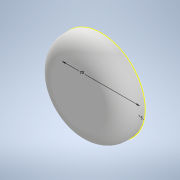
# Autodesk Inventor part: Top_and_Bottom
Saved by Autodesk Inventor 2020.2 (Build 242310000, 310)
## iProperties
Created: 2020-03-04
Part Number: Top_and_Bottom
Material: Generic
Document SubType Name: Modeling
Designer: linus
Density: 1 g/cm^3
Appearance: Default
Author: linus
Autodesk Inventor part; units mm, degrees
ref_plane "YZ Plane" through (0, 0, 0) normal (1, 0, 0) x (0, 1, 0)
ref_plane "XZ Plane" through (0, 0, 0) normal (0, 1, 0) x (-1, 0, 0)
ref_plane "XY Plane" through (0, 0, 0) normal (0, 0, 1) x (1, 0, 0)
sketch "Sketch1" plane through (0, 0, 0) normal (0, 1, 0) x (-1, 0, 0)
  line L0 (0, 0) -> (-40, 0)
  line L1 (-40, 0) -> (-40, 20)
  line L2 (-40, 20) -> (0, 20)
  line L3 (0, 20) -> (0, 0)
  dimension "d0" = 40
  dimension "d1" = 20
  constraints: 8 end point, 2 parallel, 1 horizontal, 1 perpendicular
  measures "d0" distance of L1.end L2.end
  measures "d1" distance of L0.end L1.end
revolve "Revolution1" add sketch "Sketch1" angle 360 about axis through (40, 0, 0) along (0, 0, 1)
fillet "Fillet1" radius 15 1 edges at (80, 0, 20)
sketch "Sketch2" plane through (40, 0, 0) normal (0, 0, -1) x (-1, 0, 0)
  circle A0 centre (0, 0) radius 35
  circle A1 centre (0, 0) radius 40 projected
  point P0 (40, 0)
  dimension "d4" = 70
  dimension "d5" = 5
  constraints: 1 centre point, 1 horizontal alignment
  measures "d4" diameter of A0
sketch "Sketch3" plane through (40, 0, 0) normal (0, 0, -1) x (-1, 0, 0)
  circle A0 centre (-5, 32.4685) radius 1.5
  circle A1 centre (5, 32.4685) radius 1.5
  point P0 (40, 0)
  point P1 (0, 0)
  dimension "d6" = 3
  dimension "d7" = 3
  dimension "d14" = 10
  dimension "d15" = 5
  dimension "d16" = 5
  dimension "d17" = 32.4685
  constraints: 2 centre point
  measures "d6" diameter of A0
  measures "d7" diameter of A1
  measures "d14" distance of A1.centre A0.centre
  measures "d15" horizontal distance of point (0, 0) A0.centre
  measures "d16" horizontal distance of point (0, 0) A1.centre
  measures "d17" vertical distance of point (0, 0) A0.centre
extrude "Extrusion1" cut sketch "Sketch3" against normal blind 20
sketch "Sketch4" plane through (0, 0, 0) normal (0, 1, 0) x (-1, 0, 0)
  line L0 (-40, 27.46) -> (-40, -52.54) construction
  point P0 (0, 0)
  dimension "d20" = 80
  dimension "d21" = 80
  constraints: 2 end point, 1 vertical
  measures "d20" distance of L0.start L0.end
  measures "d21" diameter of point (0, 0) L0
pattern_circular "Circular Pattern1" count 3 over 360 about axis through (40, 0, 27.46) along (0, 0, -1) of "Extrusion1"
equation "\"d6\" = d7"
body "Solid1"
